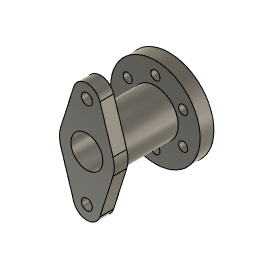
Ejercicio02_jaalobuela (Autodesk Fusion 360 design; units mm, degrees)
Autodesk Fusion 360 part; units mm, degrees
sketch "Sketch1" plane through (0, 0, 0) normal (0, 1, 0) x (1, 0, 0)
  circle A0 centre (80, -30) radius 49
  line L0 (80, -30) -> (80, -65)
  circle A1 centre (80, -65) radius 5
  circle A2 centre (110.3109, -47.5) radius 5
  circle A3 centre (110.3109, -12.5) radius 5
  circle A4 centre (80, 5) radius 5
  circle A5 centre (49.6891, -12.5) radius 5
  circle A6 centre (49.6891, -47.5) radius 5
  dimension "d1" = 98
  dimension "d3" = 10
  dimension "d5" = 360
  constraint coincident A0.centre L0.start
  constraint vertical L0
  constraint coincident L0.end A1.centre
  measures "d1" diameter of A0
  measures "d3" diameter of A1
extrude "Extrude1" add sketch "Sketch1" along normal blind 15 makes body 1
cylinder "CylinderPrimitive1" add diameter 50 height 60 placed x (1, 0, 0) y (0, 0, -1) z (0, 1, 0) at (-20, 0, 35) separate body makes body 2
move_body "Move1" bodies 2 to x (1, 0, 0) y (0, 1, 0) z (0, 0, 1) at (100, -60, -5)
sketch "Sketch3" plane through (0, 0, 0) normal (0, 1, 0) x (1, 0, 0)
  circle A0 centre (-79.5042, -85.6785) radius 6
  circle A1 centre (-79.5042, 14.3215) radius 6
  circle A2 centre (-79.5042, -35.6785) radius 17.5
  line L0 (-93.8133, -90.1785) -> (-108.1224, -44.6785)
  line L1 (-65.1951, -90.1785) -> (-50.886, -44.6785)
  line L2 (-93.8133, 18.8215) -> (-108.1224, -26.6785)
  line L3 (-65.1951, 18.8215) -> (-50.886, -26.6785)
  line L4 (-183.8133, 18.8215) -> (-198.1224, -26.6785)
  line L5 (-155.1951, 18.8215) -> (-140.886, -26.6785)
  circle A3 centre (-169.5042, -35.6785) radius 30
  circle A4 centre (-169.5042, -85.6785) radius 15
  circle A5 centre (-169.5042, -85.6785) radius 6
  circle A6 centre (-169.5042, -35.6785) radius 17.5
  circle A7 centre (-169.5042, 14.3215) radius 15
  line L6 (-155.1951, -90.1785) -> (-140.886, -44.6785)
  circle A8 centre (-169.5042, 14.3215) radius 6
  line L7 (-169.5042, -85.6785) -> (-169.5042, 14.3215)
  line L8 (-183.8133, -90.1785) -> (-198.1224, -44.6785)
  arc A9 (-93.8133, -90.1785) -> (-65.1951, -90.1785) centre (-79.5042, -85.6785) ccw
  arc A10 (-65.1951, 18.8215) -> (-93.8133, 18.8215) centre (-79.5042, 14.3215) ccw
  arc A11 (-50.886, -44.6785) -> (-50.886, -26.6785) centre (-79.5042, -35.6785) ccw
  arc A12 (-108.1224, -26.6785) -> (-108.1224, -44.6785) centre (-79.5042, -35.6785) ccw
  dimension "d10" = 100
  dimension "d11" = 12
  dimension "d12" = 12
  dimension "d13" = 30
  dimension "d14" = 30
  dimension "d15" = 35
  dimension "d16" = 60
  dimension "d17" = 100
  dimension "d18" = 12
  dimension "d19" = 12
  dimension "d20" = 30
  dimension "d21" = 30
  dimension "d22" = 35
  dimension "d23" = 60
  constraint concentric A1 A10
  constraint concentric A0 A9
  constraint concentric A2 A11
  constraint tangent L0 A11
  constraint tangent L1 A11
  constraint coincident L2.end A11
  constraint tangent L2 A11
  constraint tangent L3 A11
  constraint tangent L3 A10
  constraint tangent L2 A10
  constraint tangent L1 A9
  constraint tangent L0 A9
  constraint vertical L7
  constraint coincident A4.centre A5.centre
  constraint coincident A7.centre A8.centre
  constraint concentric A7 A8
  constraint concentric A4 A5
  constraint midpoint A3.centre L7
  constraint concentric A3 A6
  constraint coincident L8.start A4
  constraint coincident L8.end A3
  constraint tangent A3 L8
  constraint coincident L6.start A4
  constraint coincident L6.end A3
  constraint tangent A3 L6
  constraint coincident L4.start A7
  constraint coincident L4.end A3
  constraint tangent L4 A3
  constraint coincident L5.start A7
  constraint coincident L5.end A3
  constraint tangent L5 A3
  constraint tangent L5 A7
  constraint tangent L4 A7
  constraint tangent A4 L6
  constraint tangent A4 L8
  constraint concentric A11 A12
  measures "d10" distance of A0.centre A1.centre
  measures "d11" diameter of A0
  measures "d12" diameter of A1
  measures "d13" diameter of A10
  measures "d14" diameter of A9
  measures "d15" diameter of A2
  measures "d16" diameter of A11
  measures "d17" distance of A7.centre A4.centre
  measures "d18" diameter of A5
  measures "d19" diameter of A8
  measures "d20" diameter of A7
  measures "d21" diameter of A4
  measures "d22" diameter of A6
  measures "d23" diameter of A3
extrude "Extrude2" add sketch "Sketch3" along normal blind 15 separate body contours A2 | L0 L1 L2 L3 A9 A10 A11 A12 makes body 3
move_body "Move2" bodies 3 to x (1, 0, 0) y (0, 1, 0) z (0, 0, 1) at (15, 0, 0)
move_body "Move3" bodies 3 to x (1, 0, 0) y (0, 1, 0) z (0, 0, 1) at (144.5042, -75, -5.6785)
hole "Hole1" at (80, -75, 30) direction (0, 1, 0) diameter 26 depth 75 tip angle 180 counterbore diameter 35 counterbore depth 30 bodies 2 3
combine "Combine1" operation add target body 2 tool bodies 1 3
